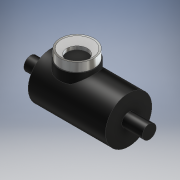
# Autodesk Inventor part: Kamera
Saved by Autodesk Inventor 2017 (Build 210142000, 142)
## iProperties
Created: 2018-08-13
Part Number: Kamera
Material: Ogólny
Document SubType Name: Modeling
Designer: Wojciech
Density: 1 g/cm^3
Appearance: Domyślna
Author: Wojciech
Autodesk Inventor part; units mm, degrees
ref_plane "YZ Plane" through (0, 0, 0) normal (1, 0, 0) x (0, 1, 0)
ref_plane "XZ Plane" through (0, 0, 0) normal (0, 1, 0) x (-1, 0, 0)
sketch "Szkic1" plane through (0, 0, 0) normal (1, 0, 0) x (0, 1, 0)
  circle A0 centre (0, 0) radius 13.5
  dimension "d0" = 27
  constraints: 1 centre point, 1 coincident
  measures "d0" diameter of A0
extrude "Wyciągnięcie proste1" add sketch "Szkic1" along normal mid plane 45
sketch "Szkic2" plane through (22.5, 0, 0) normal (1, 0, 0) x (0, 0, -1)
  circle A0 centre (0, 0) radius 4
  dimension "d3" = 8
  constraints: 1 centre point, 1 coincident
  measures "d3" diameter of A0
extrude "Wyciągnięcie proste2" add sketch "Szkic2" along normal blind 12
mirror "Odbij1" about plane through (0, 0, 0) normal (1, 0, 0) of "Wyciągnięcie proste2"
ref_plane "Płaszczyzna konstrukcyjna1" through (0, 0, 10) normal (0, 0, 1) x (1, 0, 0)
sketch "Szkic3" plane through (0, 0, 10) normal (0, 0, 1) x (1, 0, 0)
  circle A0 centre (-7.5, 0) radius 10.5
  line L0 (-22.5, 13.5) -> (-22.5, -13.5) projected
  point P0 (0, 0)
  dimension "d7" = 21
  dimension "d8" = 15
  dimension "d9" = 13.5
  constraints: 1 centre point
  measures "d7" diameter of A0
  measures "d8" distance from line of L0 A0.centre
  measures "d9" vertical distance of L0.start A0.centre
extrude "Wyciągnięcie proste3" add sketch "Szkic3" along normal blind 6
sketch "Szkic4" plane through (-7.5, 0, 16) normal (0, 0, 1) x (1, 0, 0)
  circle A0 centre (0, 0) radius 10
  line L0 (-15, 13.5) -> (-15, -13.5) projected
  circle A1 centre (0, 0) radius 6
  point P0 (7.5, 0)
  dimension "d12" = 20
  dimension "d13" = 15
  dimension "d14" = 13.5
  dimension "d15" = 12
  constraints: 2 centre point, 1 coincident
  measures "d12" diameter of A0
  measures "d13" distance from line of L0 A0.centre
  measures "d14" vertical distance of L0.start A0.centre
  measures "d15" diameter of A1
extrude "Wyciągnięcie proste4" add sketch "Szkic4" along normal blind 5
chamfer "Faza1" distance 3 angle 45 1 edges at (-13.5, 0, 21)
